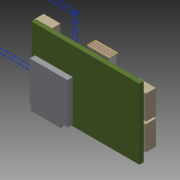
# Autodesk Inventor part: Platine
Saved by Autodesk Inventor 2014 (Build 180170000, 170)
## iProperties
Created: 2016-07-08
Part Number: Platine
Material: Generisch
Document SubType Name: Modeling
Designer: cem
Density: 1 g/cm^3
Appearance: Vorgabe
Author: cem
Autodesk Inventor part; units mm, degrees
ref_plane "YZ Plane" through (0, 0, 0) normal (1, 0, 0) x (0, 1, 0)
ref_plane "XZ Plane" through (0, 0, 0) normal (0, 1, 0) x (-1, 0, 0)
ref_plane "XY Plane" through (0, 0, 0) normal (0, 0, 1) x (1, 0, 0)
sketch "Skizze_Platine" plane through (0, 0, 0) normal (0, 1, 0) x (-1, 0, 0)
  line L0 (-20, 13) -> (20, 13)
  line L1 (20, 13) -> (20, -13)
  line L2 (20, -13) -> (-20, -13)
  line L3 (-20, -13) -> (-20, 13)
  line L4 (28, 0) -> (-28, 0) projected
  line L5 (0, -18.2) -> (0, 18.2) projected
  point P0 (0, 0)
  dimension "d0" = 40
  dimension "d1" = 26
  constraints: 8 end point, 2 parallel, 1 horizontal, 1 perpendicular, 2 other
  measures "d0" distance between parallel lines of L1 L3
  measures "d1" distance between parallel lines of L2 L0
extrude "Platine" add sketch "Skizze_Platine" along normal mid plane 1.6
sketch "Skizze2" plane through (0, 0.8, 0) normal (0, 1, 0) x (1, 0, 0)
  line L0 (-20, -13) -> (20, -13) projected
  line L1 (20, -13) -> (20, 13) projected
  line L2 (20, 13) -> (-20, 13) projected
  line L3 (-20, 13) -> (-20, -13) projected
  line L4 (-20.8, 2.6) -> (-14.6, 2.6)
  line L5 (-14.6, 2.6) -> (-14.6, -12.4)
  line L6 (-14.6, -12.4) -> (-20.8, -12.4)
  line L7 (-20.8, -12.4) -> (-20.8, 2.6)
  line L8 (-20.8, 12.4) -> (-14.6, 12.4)
  line L9 (-14.6, 12.4) -> (-14.6, 3.4)
  line L10 (-14.6, 3.4) -> (-20.8, 3.4)
  line L11 (-20.8, 3.4) -> (-20.8, 12.4)
  line L12 (14.6, 9.4) -> (20.8, 9.4)
  line L13 (20.8, 9.4) -> (20.8, 0.4)
  line L14 (20.8, 0.4) -> (14.6, 0.4)
  line L15 (14.6, 0.4) -> (14.6, 9.4)
  line L16 (14.6, -0.4) -> (20.8, -0.4)
  line L17 (20.8, -0.4) -> (20.8, -9.4)
  line L18 (20.8, -9.4) -> (14.6, -9.4)
  line L19 (14.6, -9.4) -> (14.6, -0.4)
  point P0 (0, 0)
  dimension "d4" = 15
  dimension "d5" = 0.6
  dimension "d6" = 6.2
  dimension "d7" = 0.8
  dimension "d8" = 0.6
  dimension "d9" = 9
  dimension "d14" = 3.6
  dimension "d15" = 3.6
  dimension "d17" = 0.8
  dimension "d18" = 6.2
  dimension "d19" = 9
  constraints: 32 end point, 8 parallel, 5 equal length, 4 horizontal, 4 perpendicular, 2 collinear
  measures "d4" distance between parallel lines of L6 L4
  measures "d5" distance between parallel lines of L0 L6
  measures "d6" distance between parallel lines of L5 L7
  measures "d7" distance between parallel lines of L3 L7
  measures "d8" distance between parallel lines of L8 L2
  measures "d9" distance between parallel lines of L10 L8
  measures "d14" distance between parallel lines of L12 L2
  measures "d15" distance between parallel lines of L0 L18
  measures "d17" distance between parallel lines of L1 L17
  measures "d18" distance between parallel lines of L17 L19
  measures "d19" distance between parallel lines of L14 L12
extrude "JST" add sketch "Skizze2" along normal blind 3.7 contours L6 L7 L4 L3 | L3 L4 L5 L6 | L18 L19 L16 L1 | L1 L16 L17 L18 | L10 L11 L8 L3 | L3 L8 L9 L10 | L14 L15 L12 L1 | L1 L12 L13 L14
sketch "Skizze3" plane through (0, 0.8, 0) normal (0, 1, 0) x (1, 0, 0)
  line L0 (20, 13) -> (-20, 13) projected
  line L1 (-8, 12.3) -> (-7, 12.3)
  line L2 (-7, 12.3) -> (-7, 10.6)
  line L3 (-7, 10.6) -> (-8, 10.6)
  line L4 (-8, 10.6) -> (-8, 12.3)
  line L5 (-20, 12.4) -> (-20, 3.4) projected
  line L6 (-6.5, 12.3) -> (-5.5, 12.3)
  line L7 (-5.5, 12.3) -> (-5.5, 10.6)
  line L8 (-5.5, 10.6) -> (-6.5, 10.6)
  line L9 (-6.5, 10.6) -> (-6.5, 12.3)
  line L10 (-5, 12.3) -> (-4, 12.3)
  line L11 (-4, 12.3) -> (-4, 10.6)
  line L12 (-4, 10.6) -> (-5, 10.6)
  line L13 (-5, 10.6) -> (-5, 12.3)
  point P0 (0, 0)
  dimension "d22" = 12
  dimension "d23" = 1
  dimension "d24" = 0.7
  dimension "d25" = 1.7
  dimension "d26" = 0.5
  dimension "d28" = 0.5
  constraints: 24 end point, 6 parallel, 4 equal length, 3 horizontal, 3 perpendicular, 2 collinear
  measures "d22" distance between parallel lines of L4 L5
  measures "d23" distance between parallel lines of L2 L4
  measures "d24" distance between parallel lines of L0 L1
  measures "d25" distance from line of L3 L1.start
  measures "d26" distance between parallel lines of L9 L2
  measures "d28" distance between parallel lines of L13 L7
extrude "Led" add sketch "Skizze3" along normal blind 1.1
sketch "Skizze4" plane through (0, 0.8, 0) normal (0, 1, 0) x (1, 0, 0)
  line L0 (-20, -13) -> (20, -13) projected
  line L1 (20, -13) -> (20, -9.4) projected
  line L2 (-0.5, -8.7) -> (7, -8.7)
  line L3 (7, -8.7) -> (7, -13.7)
  line L4 (7, -13.7) -> (-0.5, -13.7)
  line L5 (-0.5, -13.7) -> (-0.5, -8.7)
  point P0 (0, 0)
  dimension "d31" = 5
  dimension "d33" = 20.5
  dimension "d34" = 7.5
  dimension "d35" = 4.3
  constraints: 8 end point, 2 parallel, 1 horizontal, 1 perpendicular
  measures "d31" distance between parallel lines of L4 L2
  measures "d33" distance between parallel lines of L1 L5
  measures "d34" distance between parallel lines of L3 L5
  measures "d35" distance between parallel lines of L0 L2
extrude "USB" add sketch "Skizze4" along normal blind 2.8
ref_plane "Arbeitsebene1" through (-0.5, 0.8, 14.3) normal (0, 0, 1) x (1, 0, 0)
sketch "Skizze6" plane through (-0.5, 0.8, 14.3) normal (0, 0, 1) x (1, 0, 0)
  line L0 (7.5, 0) -> (0, 0) projected
  line L1 (7.5, 0) -> (7.5, 2.8) projected
  line L2 (0, 2.8) -> (7.5, 2.8) projected
  line L3 (0, 0) -> (0, 2.8) projected
  line L4 (-1.3807, 1.4) -> (9.761, 1.4) construction
  line L5 (3.75, 4.4264) -> (3.75, -1.3198) construction
  line L6 (-0.2, 3.1) -> (7.7, 3.1)
  line L7 (7.7, 3.1) -> (7.7, -0.3)
  line L8 (7.7, -0.3) -> (-0.2, -0.3)
  line L9 (-0.2, -0.3) -> (-0.2, 3.1)
  point P0 (0.5, -0.8)
  dimension "d42" = 0.2
  dimension "d43" = 0.3
  constraints: 12 end point, 3 perpendicular, 2 parallel, 1 horizontal, 2 other
  measures "d42" distance between parallel lines of L3 L9
  measures "d43" distance between parallel lines of L2 L6
loft "Erhebung1" add profiles "Skizze6" separate body section 1 edges at (3.25, 0.8, 13.7) (7, 2.2, 13.7) (3.25, 3.6, 13.7) (-0.5, 2.2, 13.7) contours L0 L3 L2 L1 | L6 L7 L8 L9
sketch "Skizze7" plane through (0, -0.8, 0) normal (0, -1, 0) x (1, 0, 0)
  line L0 (-20, 13) -> (-20, -13) projected
  line L1 (-20, -13) -> (20, -13) projected
  line L2 (-18.7, 2.8) -> (-4.7, 2.8)
  line L3 (-4.7, 2.8) -> (-4.7, -12.4)
  line L4 (-4.7, -12.4) -> (-18.7, -12.4)
  line L5 (-18.7, -12.4) -> (-18.7, 2.8)
  line L6 (-18.7, -11.4) -> (-7.2, -11.4)
  line L7 (-7.2, -11.4) -> (-7.2, -12.4)
  line L8 (-7.2, -12.4) -> (-18.7, -12.4)
  line L9 (-18.7, -12.4) -> (-18.7, -11.4)
  point P0 (0, 0)
  dimension "d48" = 1.3
  dimension "d49" = 0.6
  dimension "d50" = 14
  dimension "d51" = 15.2
  dimension "d52" = 1
  dimension "d53" = 2.5
  constraints: 16 end point, 4 parallel, 2 horizontal, 2 perpendicular, 2 point on line
  measures "d48" distance between parallel lines of L5 L0
  measures "d49" distance between parallel lines of L1 L4
  measures "d50" distance between parallel lines of L3 L5
  measures "d51" distance between parallel lines of L4 L2
  measures "d52" distance between parallel lines of L8 L6
  measures "d53" distance between parallel lines of L3 L7
extrude "Slot" add sketch "Skizze7" along normal blind 1.95 contours L2 L3 L4 L7 L6 L5 bodies 1
sketch "Skizze8" plane through (-7.2, -0.8, -11.4) normal (0, 0, -1) x (-1, 0, 0)
  line L0 (0, 0) -> (11.5, 0) projected
  line L1 (0, 0) -> (0, -1.95) projected
  line L2 (11.5, -1.95) -> (0, -1.95) projected
  line L3 (0.2, -0.8) -> (11.3, -0.8)
  line L4 (11.3, -0.8) -> (11.3, -1.8)
  line L5 (11.3, -1.8) -> (0.2, -1.8)
  line L6 (0.2, -1.8) -> (0.2, -0.8)
  line L7 (5.75, 0.6662) -> (5.75, -3.1809) construction
  point P0 (-7.2, 0.8)
  dimension "d56" = 0.8
  dimension "d57" = 1
  dimension "d58" = 0.2
  constraints: 10 end point, 2 parallel, 2 perpendicular, 1 horizontal, 1 other
  measures "d56" distance between parallel lines of L3 L0
  measures "d57" distance between parallel lines of L5 L3
  measures "d58" distance between parallel lines of L6 L1
extrude "Card" add sketch "Skizze8" along normal blind 2.6 bodies 1
